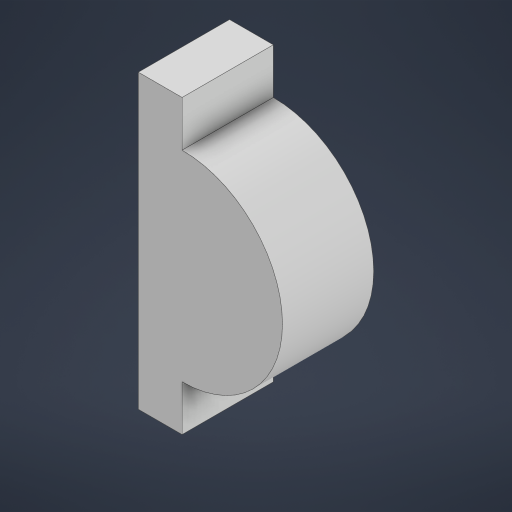
# Autodesk Inventor part: ChargeLED
Saved by Autodesk Inventor 2023 (Build 270158000, 158)
## iProperties
Created: 2022-10-27
Part Number: ChargeLED
Material: Generic
Document SubType Name: Modeling
Designer: jevan
Density: 1 g/cm^3
Appearance: Default
Author: jevan
Autodesk Inventor part; units mm, degrees
ref_plane "YZ Plane" through (0, 0, 0) normal (1, 0, 0) x (0, 1, 0)
ref_plane "XZ Plane" through (0, 0, 0) normal (0, 1, 0) x (-1, 0, 0)
ref_plane "XY Plane" through (0, 0, 0) normal (0, 0, 1) x (1, 0, 0)
sketch "Sketch1" plane through (0, 0, 0) normal (0, 0, 1) x (1, 0, 0)
  line L0 (0, 0) -> (0.48, 0)
  line L1 (0.48, -3.2) -> (0, -3.2)
  line L2 (0, -3.2) -> (0, 0)
  arc A0 (0.48, -2.7) -> (0.48, -0.5) centre (0.48, -1.6) ccw
  line L3 (0.48, 0) -> (0.48, -0.5)
  line L4 (0.48, -2.7) -> (0.48, -3.2)
  line L5 (0, -1.6) -> (0.48, -1.6)
  dimension "d0" = 0.48
  dimension "d1" = 3.2
  dimension "d7" = 2.2
  constraints: 12 end point, 3 parallel, 2 horizontal, 2 perpendicular, 2 point on circle, 1 centre point, 1 collinear, 1 line through centre, 1 midpoint
  measures "d0" distance of L1.start L1.end
  measures "d1" distance of L0.end L1.start
  measures "d7" diameter of A0
extrude "Extrusion1" add sketch "Sketch1" along normal blind 1
body "Solid1"
